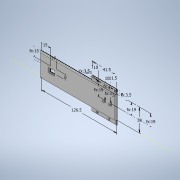
# Autodesk Inventor part: roof
Saved by Autodesk Inventor 2020 (Build 240168000, 168)
## iProperties
Created: 2022-09-29
Part Number: roof
Material: 일반
Document SubType Name: Modeling
Designer: taewo
Density: 1 g/cm^3
Appearance: 기본값
Author: taewo
Autodesk Inventor part; units mm, degrees
ref_plane "YZ Plane" through (0, 0, 0) normal (1, 0, 0) x (0, 1, 0)
ref_plane "XZ Plane" through (0, 0, 0) normal (0, 1, 0) x (-1, 0, 0)
ref_plane "XY Plane" through (0, 0, 0) normal (0, 0, 1) x (1, 0, 0)
sketch "sketch" plane through (0, 0, 0) normal (0, 0, 1) x (1, 0, 0)
  line L0 (-52.714, 0) -> (218.2838, 0) construction
  line L1 (0, -17.4) -> (0, 55.4) construction
  line L2 (0, 38) -> (126.5, 38)
  line L3 (126.5, 38) -> (126.5, 0)
  line L4 (126.5, 0) -> (0, 0)
  line L5 (0, 0) -> (0, 38)
  line L6 (15, 23) -> (25, 23)
  line L7 (25, 23) -> (25, 15)
  line L8 (25, 15) -> (15, 15)
  line L9 (15, 15) -> (15, 23)
  circle A0 centre (116.5, 19) radius 1.5
  circle A1 centre (106.5, 19) radius 1.5
  line L10 (85, 45) -> (126.5, 45)
  line L11 (126.5, 45) -> (126.5, 38)
  line L12 (126.5, 38) -> (85, 38)
  line L13 (85, 38) -> (85, 45)
  line L14 (-14, 19) -> (179.5698, 19) construction
  circle A2 centre (95, 41.5) radius 1.5
  circle A3 centre (115, 41.5) radius 1.5
  line L15 (85, -7) -> (126.5, -7)
  line L16 (126.5, -7) -> (126.5, 0)
  line L17 (85, 0) -> (85, -7)
  circle A4 centre (95, -3.5) radius 1.5
  circle A5 centre (115, -3.5) radius 1.5
  dimension "d0" = 126.5
  dimension "d1" = 38
  dimension "d2" = 15
  dimension "d3" = 10
  dimension "d4" = 8
  dimension "d5" = 15
  dimension "d6" = 3
  dimension "d7" = 10
  dimension "d8" = 3
  dimension "d9" = 10
  dimension "d10" = 19
  dimension "d11" = 19
  dimension "d12" = 41.5
  dimension "d13" = 7
  dimension "d14" = 19
  dimension "d15" = 10
  dimension "d16" = 11.5
  dimension "d17" = 3
  dimension "d18" = 3
  dimension "d19" = 3.5
  dimension "d20" = 3.5
  constraints: 32 end point, 6 centre point, 6 parallel, 5 symmetric about line, 4 horizontal, 3 perpendicular, 2 other
  measures "d0" distance of L4.end L3.end
  measures "d1" distance of L2.end L3.end
  measures "d2" distance between parallel lines of L5 L9
  measures "d3" distance of L6.start L6.end
  measures "d4" distance of L6.end L7.end
  measures "d5" distance between parallel lines of L2 L6
  measures "d6" diameter of A0
  measures "d7" distance from line of L3 A0.centre
  measures "d8" diameter of A1
  measures "d9" distance of A0.centre A1.centre
  measures "d10" distance from line of L2 A0.centre
  measures "d11" distance from line of L2 A1.centre
  measures "d12" distance of L10.start L10.end
  measures "d13" distance of L10.end L2.end
  measures "d14" distance between parallel lines of L14 L2
  measures "d15" distance from line of L13 A2.centre
  measures "d16" distance from line of L11 A3.centre
  measures "d17" diameter of A2
  measures "d18" diameter of A3
  measures "d19" distance from line of L2 A2.centre
  measures "d20" distance from line of L2 A3.centre
extrude "roof" add sketch "sketch" along normal blind 3 contours L2 L3 L4 L5
extrude "bolt" add sketch "sketch" along normal blind 1.5 contours L13 L10 L11 L2 | L4 L16 L15 L17
fillet "so_hurt" radius 1 10 edges at (63.25, 38, 3) (63.25, 0, 3) (126.5, 19, 3) (85, -3.5, 1.5) (105.75, -7, 1.5) (126.5, 41.5, 1.5) (105.75, 45, 1.5) (85, 41.5, 1.5) (0, 19, 3) (126.5, -3.5, 1.5)
equation "\"d8\" = d6"
equation "\"d10\" = 0.5 * d1"
equation "\"d11\" = 0.5 * d1"
equation "\"d14\" = 0.5 * d1"
equation "\"d17\" = d6"
equation "\"d18\" = d6"
equation "\"d19\" = 0.5 * d13"
equation "\"d20\" = 0.5 * d13"
